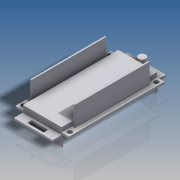
# Autodesk Inventor part: 76608-White
Saved by Autodesk Inventor 2016 SP2 (Build 200236200, 236)
## iProperties
Created: 2015-08-26
Part Number: 76608-White
Material: ABS Plastic
Document SubType Name: Modeling
Designer: D. Kohfeld
Density: 1.06 g/cm^3
Appearance: White
Mass: 4.70679 g
Surface Area: 65.2492 cm^2
Volume: 4.44037 cm^3
Author: D. Kohfeld
Autodesk Inventor part; units mm, degrees
ref_plane "YZ Plane" through (0, 0, 0) normal (1, 0, 0) x (0, 1, 0)
ref_plane "XZ Plane" through (0, 0, 0) normal (0, 1, 0) x (-1, 0, 0)
ref_plane "XY Plane" through (0, 0, 0) normal (0, 0, 1) x (1, 0, 0)
sketch "Sketch2" plane through (0, 0, 0) normal (0, 1, 0) x (-1, 0, 0)
  line L0 (-14.4, 25.6) -> (14.4, 25.6)
  line L1 (14.4, 25.6) -> (14.4, -25.6)
  line L2 (14.4, -25.6) -> (-14.4, -25.6)
  line L3 (-14.4, -25.6) -> (-14.4, 25.6)
  line L4 (10.4, 25.6) -> (10.4, -25.6)
  line L5 (-10.4, 25.6) -> (-10.4, -25.6)
  line L6 (-11.2, 20) -> (-12, 20)
  line L7 (-12, 20) -> (-12, -20)
  line L8 (-12, -20) -> (-11.2, -20)
  line L9 (-11.2, -20) -> (-11.2, 20)
  line L10 (11.2, 20) -> (12, 20)
  line L11 (12, 20) -> (12, -20)
  line L12 (12, -20) -> (11.2, -20)
  line L13 (11.2, -20) -> (11.2, 20)
  line L14 (-10.4, 25.6) -> (10.4, -25.6) construction
  line L15 (-11.2, 20) -> (11.2, -20) construction
  circle A0 centre (12.4, 23.2) radius 1.2
  circle A1 centre (-12.4, 23.2) radius 1.2
  circle A2 centre (-12.4, -23.2) radius 1.2
  circle A3 centre (12.4, -23.2) radius 1.2
  line L16 (-12.4, 23.2) -> (12.4, 23.2) construction
  line L17 (-12.4, 23.2) -> (-12.4, -23.2) construction
  point P0 (0, 0)
  point P1 (0, 25.6)
  point P2 (-14.4, 0)
  point P3 (0, 23.2)
  point P4 (0, 0)
  point P5 (-12.4, 0)
  dimension "d0" = 28.8
  dimension "d1" = 51.2
  dimension "d2" = 20.8
  dimension "d3" = 22.4
  dimension "d4" = 0.8
  dimension "d5" = 40
  dimension "d6" = 2.4
  dimension "d7" = 46.4
  dimension "d8" = 24.8
  constraints: 36 end point, 7 midpoint, 6 parallel, 4 centre point, 4 horizontal, 4 horizontal alignment, 4 point on line, 3 equal radius, 3 perpendicular, 3 vertical, 3 vertical alignment, 2 equal length
  measures "d0" distance of L0.start L0.end
  measures "d1" distance of L2.end L0.start
  measures "d2" distance between parallel lines of L5 L4
  measures "d3" distance between parallel lines of L9 L13
  measures "d4" distance between parallel lines of L13 L11
  measures "d5" distance of L6.end L7.end
  measures "d6" diameter of A3
  measures "d7" distance of L16.start L17.end
  measures "d8" distance from line of A3.centre L17
extrude "Extrusion1" add sketch "Sketch2" against normal blind 1.2 contours L0 L5 L2 L3 | L0 L4 L2 L5 | L0 L1 L2 L4 | L9 L8 L7 L6 | L10 L11 L12 L13
extrude "Extrusion2" add sketch "Sketch2" along normal blind 2.4 contours L0 L4 L2 L5
extrude "Extrusion3" add sketch "Sketch2" along normal blind 10.8 contours L9 L8 L7 L6 | L10 L11 L12 L13
sketch "Sketch3" plane through (0, 0, 0) normal (1, 0, 0) x (0, 1, 0)
  line L0 (-1.2, -25.6) -> (-1.2, 25.6) projected
  line L1 (-1.2, 25.6) -> (-1.2, 30.4)
  line L2 (-1.2, 30.4) -> (-2.4, 30.4)
  line L3 (-2.4, 30.4) -> (-2.4, 26)
  line L4 (-2.4, 26) -> (-6.4, 26)
  line L5 (-6.4, 26) -> (-7.6, 24.8)
  line L6 (-7.6, 24.8) -> (-2, 24.8)
  line L7 (-2, 24.8) -> (-2, -24.8)
  line L8 (-2, -24.8) -> (-7.6, -24.8)
  line L9 (-7.6, -24.8) -> (-6.4, -26)
  line L10 (-6.4, -26) -> (-2.4, -26)
  line L11 (-2.4, -26) -> (-2.4, -30.4)
  line L12 (-2.4, -30.4) -> (-1.2, -30.4)
  line L13 (-1.2, -30.4) -> (-1.2, -25.6)
  point P0 (0, 0)
  point P1 (-2, 0)
  point P2 (-1.2, 0)
  dimension "d15" = 1.2
  dimension "d16" = 4.8
  dimension "d17" = 4.4
  dimension "d18" = 4
  dimension "d19" = 1.2
  dimension "d20" = 5.2
  dimension "d21" = 0.4
  constraints: 26 end point, 6 horizontal, 5 equal length, 5 vertical, 2 midpoint, 1 horizontal alignment
  measures "d15" distance between parallel lines of L1 L3
  measures "d16" distance from line of L2 L0.end
  measures "d17" distance between parallel lines of L4 L2
  measures "d18" distance of L3.end L4.end
  measures "d19" distance between parallel lines of L6 L4
  measures "d20" distance from line of L5.end L3
  measures "d21" distance between parallel lines of L7 L3
extrude "Extrusion4" add sketch "Sketch3" against normal up to surface (20.8 mm away) from surface at 10.4
sketch "Sketch4" plane through (-10.4, -2.4, -30.4) normal (0, -1, 0) x (1, 0, 0)
  line L0 (0, 0) -> (20.8, 0) projected
  line L1 (0, 4.4) -> (20.8, 4.4) projected
  line L2 (0, 60.8) -> (0, 56.4) projected
  line L3 (0, 56.4) -> (20.8, 56.4) projected
  line L4 (20.8, 56.4) -> (20.8, 60.8) projected
  line L5 (0, 60.8) -> (20.8, 60.8) projected
  line L6 (8.4, 4.4) -> (9.2, 5.2)
  line L7 (9.2, 5.2) -> (11.6, 5.2)
  line L8 (11.6, 5.2) -> (12.4, 4.4)
  circle A0 centre (10.4, 2.4) radius 2
  circle A1 centre (10.4, 2.4) radius 1.2
  line L9 (14.8, 57.2) -> (6, 57.2)
  line L10 (6, 57.2) -> (6, 59.6)
  line L11 (6, 59.6) -> (14.8, 59.6)
  line L12 (14.8, 59.6) -> (14.8, 57.2)
  point P0 (10.4, 30.4)
  point P1 (10.4, 5.2)
  point P2 (10.4, 4.4)
  point P3 (10.4, 57.2)
  point P4 (10.4, 56.4)
  dimension "d24" = 2.4
  dimension "d25" = 8.8
  dimension "d26" = 0.8
  dimension "d27" = 4
  dimension "d28" = 2.4
  dimension "d29" = 0.8
  dimension "d30" = 4
  dimension "d31" = 2.4
  dimension "d32" = 2.4
  constraints: 14 end point, 4 midpoint, 3 vertical alignment, 2 centre point, 2 horizontal, 2 parallel, 2 perpendicular, 2 point on line, 1 coincident
  measures "d24" distance of L9.end L10.end
  measures "d25" distance of L10.end L11.end
  measures "d26" distance between parallel lines of L3 L9
  measures "d27" distance of L6.start L8.end
  measures "d28" distance of L6.end L7.end
  measures "d29" distance between parallel lines of L1 L7
  measures "d30" diameter of A0
  measures "d31" diameter of A1
  measures "d32" distance from line of A0.centre L0
extrude "Extrusion5" cut sketch "Sketch4" against normal through all contours L9 L10 L11 L12
extrude "Extrusion6" cut sketch "Sketch4" along normal through all contours L6 L7 L8 L1
extrude "Extrusion7" add sketch "Sketch4" along normal blind 0.8 contours A0
extrude "Extrusion8" add sketch "Sketch4" against normal blind 5.6 contours A0 | A1
extrude "Extrusion9" cut sketch "Sketch4" against normal blind 4.4 contours A1
sketch "Sketch5" plane through (0, 0, 0) normal (0, 0, 1) x (1, 0, 0)
  line L0 (-10.4, -2) -> (10.4, -2) projected
  line L1 (-0.4, -2) -> (0.4, -2)
  line L2 (0.4, -2) -> (1.6763, -0.7246)
  line L3 (-0.4, -2) -> (-1.6763, -0.7246)
  arc A0 (-1.6763, -0.7246) -> (-9.1237, -0.7246) centre (-5.4, -4.451) ccw
  line L4 (-9.1237, -0.7246) -> (-10.4, -2)
  arc A1 (9.1237, -0.7246) -> (1.6763, -0.7246) centre (5.4, -4.451) ccw
  line L5 (9.1237, -0.7246) -> (10.4, -2)
  line L6 (-5.4, -4.451) -> (5.4, -4.451) construction
  point P0 (0, 0)
  point P1 (0, -2)
  point P2 (0, -2)
  point P3 (0, -4.451)
  dimension "d43" = 10.8
  dimension "d44" = 0.8
  dimension "d45" = 2.817
  dimension "d46" = 5.268
  constraints: 12 end point, 4 point on circle, 4 tangent, 3 midpoint, 2 centre point, 2 point on line, 1 coincident, 1 equal radius, 1 horizontal, 1 horizontal alignment, 1 vertical alignment
  measures "d43" distance of L6.end L6.start
  measures "d44" distance of L1.start L1.end
  measures "d45" distance edge to line of A0 L0
  measures "d46" radius of A0
extrude "Extrusion10" cut sketch "Sketch5" against normal up to surface (49.6 mm away) from surface at 24.8
chamfer "Chamfer1" distance 0.6 distance2 0.8 1 edges at (-1.2, -3.2, -28) measured on face at (-1.7, -3.2, -28)
fillet "Fillet1" radius 0.1 100 edges at (-12, 5.4, 20) (-11.2, 5.4, 20) (-11.6, 10.8, 20) (-12, 10.8, 0) (-11.2, 10.8, 0) (-11.2, 5.4, -20) (-12, 5.4, -20) (-11.6, 10.8, -20) (11.2, 5.4, 20) (12, 5.4, 20) (11.6, 10.8, 20) (11.2, 10.8, 0) (12, 10.8, 0) (12, 5.4, -20) (11.6, 10.8, -20) (11.2, 5.4, -20) (10.4, 2.4, 0) (10.4, 1.2, 25.6) (0, 2.4, 25.6) (-10.4, 1.2, 25.6) (-10.4, 2.4, 0) (-10.4, 1.2, -25.6) (0, 2.4, -25.6) (10.4, 1.2, -25.6) (12.4, 0, -25.6) (14.4, -0.6, -25.6) (14.4, -1.2, 0) (12.4, -1.2, -25.6) (14.4, 0, 0) (14.4, -0.6, 25.6) (12.4, 0, 25.6) (12.4, -1.2, 25.6) (-12.4, -1.2, 25.6) (-12.4, 0, 25.6) (-14.4, -0.6, 25.6) (-14.4, 0, 0) (-14.4, -1.2, 0) (-14.4, -0.6, -25.6) (-12.4, 0, -25.6) (-12.4, -1.2, -25.6) (10.4, -1.2, 28) (10.4, -2.4, 28.2) (10.4, -1.8, 30.4) (0, -1.2, 30.4) (0, -2.4, 30.4) (-10.4, -1.8, 30.4) (-10.4, -2.4, 28.2) (-10.4, -1.2, 28) (-4.4, -1.2, 28) (0, -1.2, 29.2) (0, -1.2, 26.8) (4.4, -1.2, 28) (4.4, -2.4, 28) (0, -2.4, 29.2) (-4.4, -2.4, 28) (0, -2.4, 26.8) (-10.4, -1.2, -28) (-10.4, -2.4, -28.2) (-10.4, -1.8, -30.4) (0, -1.2, -30.4) (0, -2.4, -30.4) (10.4, -1.8, -30.4) (-2, 3.2, -28) (10.4, -1.2, -28) (10.4, -2.4, -28.2) (10.4, -2, 0) (10.4, -4.8, 24.8) (10.4, -7, 25.4) (0, -7.6, 24.8) (0, -6.4, 26) (10.4, -4.4, 26) (-10.4, -7, 25.4) (-10.4, -4.4, 26) (-10.4, -4.8, 24.8) (-10.4, -2, 0) (0.4, -2, 0) (-0.4, -2, 0) (10.4, -4.8, -24.8) (10.4, -4.4, -26) (10.4, -7, -25.4) (6.2, -6.4, -26) (0, -7.6, -24.8) (-6.2, -6.4, -26) (-10.4, -7, -25.4) (-10.4, -4.4, -26) (-10.4, -4.8, -24.8) (-2, -3.2, -28) (-2, -4.4, -26) (-1.6, -6.8, -25.6) (0, -7.2, -25.2) (1.6, -6.8, -25.6) (2, -4.4, -26) (13.6, -1.2, -23.2) (13.6, 0, -23.2) (-11.2, -1.2, -23.2) (-11.2, 0, -23.2) (13.6, -1.2, 23.2) (13.6, 0, 23.2) (-11.2, -1.2, 23.2) (-11.2, 0, 23.2)
body "Solid1"
